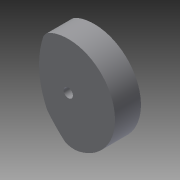
# Autodesk Inventor part: STOPPER 3.0 ish
Saved by Autodesk Inventor 2015 (Build 190159000, 159)
## iProperties
Created: 2016-02-18
Part Number: STOPPER 3.0 ish
Material: Generic
Document SubType Name: Modeling
Designer: JovinHo
Density: 1 g/cm^3
Appearance: Default
Author: JovinHo
Autodesk Inventor part; units mm, degrees
ref_plane "YZ Plane" through (0, 0, 0) normal (1, 0, 0) x (0, 1, 0)
ref_plane "XZ Plane" through (0, 0, 0) normal (0, 1, 0) x (-1, 0, 0)
ref_plane "XY Plane" through (0, 0, 0) normal (0, 0, 1) x (1, 0, 0)
sketch "Sketch1" plane through (0, 0, 0) normal (0, 0, 1) x (1, 0, 0)
  circle A0 centre (0, 0) radius 45.72
  dimension "d0" = 91.44
  constraints: 1 centre point, 1 coincident
  measures "d0" diameter of A0
extrude "Extrusion1" add sketch "Sketch1" along normal blind 25.4
sketch "Sketch2" plane through (0, 0, 25.4) normal (0, 0, 1) x (1, 0, 0)
  line L0 (-0.3558, -0.3558) -> (-20.8252, -24.6266)
  circle A0 centre (0, 0) radius 45.72 projected
  arc A1 (-23.0314, 39.4952) -> (-20.8252, -24.6266) centre (52.3824, 9.9911) ccw
  arc A2 (-20.8252, -24.6266) -> (0, -45.72) centre (78.7583, 52.8636) ccw
  dimension "d4" = 31.75
  constraints: 6 point on circle, 2 centre point, 2 end point
  measures "d4" distance of L0.start L0.end
extrude "Extrusion2" cut sketch "Sketch2" against normal through all contours A1 A2 A0 picked at (-31.6605, -11.4732)
sketch "Sketch3" plane through (0, 0, 25.4) normal (0, 0, 1) x (1, 0, 0)
  arc A0 (-18.5763, 41.5522) -> (-25.0291, 34.3173) centre (-12.3609, 29.5137) ccw
  point P0 (0, 0)
  constraints: 2 point on circle, 1 centre point
extrude "Extrusion3" cut sketch "Sketch3" against normal through all fills toward (-22.5093, 38.565) open curves A0
sketch "Sketch5" plane through (0, 0, 25.4) normal (0, 0, 1) x (1, 0, 0)
  arc A0 (-6.0617, -41.7478) -> (9.5815, -44.6809) centre (5.7004, -22.198) ccw
  point P0 (0, 0)
  constraints: 2 point on circle, 1 centre point
extrude "Extrusion4" cut sketch "Sketch5" against normal through all fills toward (1.4866, -44.6718) open curves A0
sketch "Sketch6" plane through (0, 0, 25.4) normal (0, 0, 1) x (1, 0, 0)
  circle A0 centre (0, 0) radius 4.572
  dimension "d13" = 9.144
  constraints: 1 centre point, 1 coincident
  measures "d13" diameter of A0
extrude "Extrusion5" cut sketch "Sketch6" against normal through all
body "Solid1"
